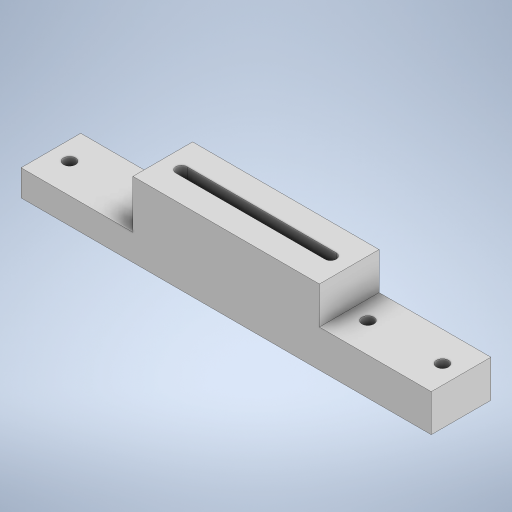
# Autodesk Inventor part: middle_hole
Saved by Autodesk Inventor 2023.1 (Build 271208000, 208)
## iProperties
Created: 2023-11-20
Part Number: middle_hole
Material: Všeobecné
Document SubType Name: Modeling
Designer: zavrel
Density: 1 g/cm^3
Appearance: Výchozí
Author: zavrel
Autodesk Inventor part; units mm, degrees
ref_plane "YZ Plane" through (0, 0, 0) normal (1, 0, 0) x (0, 1, 0)
ref_plane "XZ Plane" through (0, 0, 0) normal (0, 1, 0) x (-1, 0, 0)
ref_plane "XY Plane" through (0, 0, 0) normal (0, 0, 1) x (1, 0, 0)
sketch "Náčrt1" plane through (0, 0, 0) normal (0, 1, 0) x (-1, 0, 0)
  line L0 (0, 0) -> (110, 0)
  line L1 (110, 0) -> (110, -16)
  line L2 (110, -16) -> (0, -16)
  line L3 (0, -16) -> (0, 0)
  line L4 (55, -16) -> (55, 0) construction
  line L5 (110, -8) -> (0, -8) construction
  circle A0 centre (105, -8) radius 1.6
  circle A1 centre (85, -8) radius 1.6
  line L6 (105, -8) -> (105, -2.8731) construction
  line L7 (85, -8) -> (85, -2.8731) construction
  line L8 (105, -5.7373) -> (103.8686, -6.8686)
  line L9 (105, -5.7373) -> (106.1314, -6.8686)
  line L10 (85, -5.7373) -> (83.8686, -6.8686)
  line L11 (85, -5.7373) -> (86.1314, -6.8686)
  circle A2 centre (5, -8) radius 1.6
  circle A3 centre (25, -8) radius 1.6
  line L12 (5, -8) -> (5, -2.8731) construction
  line L13 (25, -8) -> (25, -2.8731) construction
  line L14 (5, -5.7373) -> (6.1314, -6.8686)
  line L15 (5, -5.7373) -> (3.8686, -6.8686)
  line L16 (25, -5.7373) -> (26.1314, -6.8686)
  line L17 (25, -5.7373) -> (23.8686, -6.8686)
  dimension "d0" = 16
  dimension "d1" = 110
  dimension "d4" = 3.2
  dimension "d6" = 25
  dimension "d7" = 5
  dimension "d49" = 90
  dimension "d54" = 90
  constraints: 36 end point, 10 symmetric about line, 4 centre point, 4 midpoint, 4 point on circle, 4 point on line, 2 parallel, 2 tangent, 2 vertical, 1 equal radius, 1 horizontal, 1 perpendicular, 2 other
  measures "d0" distance between parallel lines of L2 L0
  measures "d1" distance of L1.end L2.end
  measures "d4" diameter of A0
  measures "d6" distance from line of L1 L7.start
  measures "d7" distance from line of L1 L6.start
  measures "d49" angle of L9 L8
  measures "d54" angle of L11 L10
extrude "Vysunutí1" add sketch "Náčrt1" along normal blind 20 contours L0 L1 L2 L3 | A0 L8 L9 | A1 L10 L11 | A2 L15 L14 | A3 L17 L16
sketch "Sketch11" plane through (0, 20, 0) normal (0, 1, 0) x (1, 0, 0)
  line L0 (0, 16) -> (-110, 16) projected
  line L1 (-110, 16) -> (-110, 0) projected
  line L2 (-110, 0) -> (0, 0) projected
  line L3 (0, 0) -> (0, 16) projected
  circle A0 centre (-5, 8) radius 1.6 projected
  circle A1 centre (-25, 8) radius 1.6 projected
  circle A2 centre (-85, 8) radius 1.6 projected
  circle A3 centre (-105, 8) radius 1.6 projected
  line L4 (-30, 16) -> (-30, 0)
  line L5 (-110, 0) -> (0, 0) projected
  dimension "d55" = 30
  constraints: 2 end point, 2 point on line, 1 perpendicular
  measures "d55" distance between parallel lines of L3 L4
extrude "Extrusion9" cut sketch "Sketch11" against normal blind 10 contours L3 L2 L4 L0 | A0 | A1
sketch "Sketch12" plane through (0, 20, 0) normal (0, 1, 0) x (1, 0, 0)
  circle A0 centre (-105, 8) radius 1.6 projected
  circle A1 centre (-85, 8) radius 1.6 projected
  line L0 (-30, 0) -> (-30, 16) projected
  line L1 (-30, 16) -> (-110, 16) projected
  line L2 (-110, 16) -> (-110, 0) projected
  line L3 (-110, 0) -> (-30, 0) projected
  line L4 (0, 16) -> (-110, 16) projected
  line L5 (-80, 16) -> (-80, 0)
  line L6 (-110, 0) -> (0, 0) projected
  dimension "d58" = 30
  constraints: 2 end point, 2 point on line, 1 perpendicular
  measures "d58" distance between parallel lines of L5 L2
extrude "Extrusion10" cut sketch "Sketch12" against normal blind 13 contours A0 | A1 | L3 L2 L1 L5
sketch "Sketch13" plane through (0, 0, 0) normal (0, -1, 0) x (1, 0, 0)
  line L0 (0, -16) -> (-110, -16) projected
  line L1 (0, 0) -> (0, -16) projected
  line L2 (-110, 0) -> (0, 0) projected
  line L3 (-110, -16) -> (-110, 0) projected
  circle A0 centre (-5, -8) radius 1.6 projected
  circle A1 centre (-25, -8) radius 1.6 projected
  circle A2 centre (-85, -8) radius 1.6 projected
  circle A3 centre (-105, -8) radius 1.6 projected
  line L4 (-110, -16) -> (-110, 0) construction
  line L5 (-110, -8) -> (0, -8) construction
  line L6 (-75, -8) -> (-35, -8) construction
  line L7 (-75, -9.5) -> (-35, -9.5)
  line L8 (-35, -6.5) -> (-75, -6.5)
  arc A4 (-75, -6.5) -> (-75, -9.5) centre (-75, -8) ccw
  arc A5 (-35, -9.5) -> (-35, -6.5) centre (-35, -8) ccw
  point P0 (-55, -8)
  dimension "d61" = 3
  dimension "d62" = 40
  constraints: 10 end point, 4 midpoint, 4 point on circle, 4 tangent, 2 centre point, 1 parallel, 1 point on line
  measures "d61" distance between parallel lines of L7 L8
  measures "d62" distance of L6.start L6.end
extrude "Extrusion11" cut sketch "Sketch13" against normal through all contours A4 L8 A5 L7
sketch "Sketch14" plane through (0, 0, 0) normal (0, -1, 0) x (1, 0, 0)
  line L0 (-75, -6.5) -> (-35, -6.5) projected
  arc A0 (-35, -9.5) -> (-35, -6.5) centre (-35, -8) ccw projected
  line L1 (-35, -9.5) -> (-75, -9.5) projected
  arc A1 (-75, -6.5) -> (-75, -9.5) centre (-75, -8) ccw projected
  line L2 (0, -16) -> (-110, -16) projected
  line L3 (0, 0) -> (0, -16) projected
  line L4 (-110, 0) -> (0, 0) projected
  line L5 (-110, -16) -> (-110, 0) projected
  circle A2 centre (-5, -8) radius 1.6 projected
  circle A3 centre (-25, -8) radius 1.6 projected
  circle A4 centre (-85, -8) radius 1.6 projected
  circle A5 centre (-105, -8) radius 1.6 projected
  circle A6 centre (-105, -8) radius 1.6 projected
  line L6 (-101.8246, -8) -> (-103.4123, -10.75)
  line L7 (-103.4123, -10.75) -> (-106.5877, -10.75)
  line L8 (-106.5877, -10.75) -> (-108.1754, -8)
  line L9 (-108.1754, -8) -> (-106.5877, -5.25)
  line L10 (-106.5877, -5.25) -> (-103.4123, -5.25)
  line L11 (-103.4123, -5.25) -> (-101.8246, -8)
  line L12 (-81.8246, -8) -> (-83.4123, -10.75)
  line L13 (-83.4123, -10.75) -> (-86.5877, -10.75)
  line L14 (-86.5877, -10.75) -> (-88.1754, -8)
  line L15 (-88.1754, -8) -> (-86.5877, -5.25)
  line L16 (-86.5877, -5.25) -> (-83.4123, -5.25)
  line L17 (-83.4123, -5.25) -> (-81.8246, -8)
  line L18 (-21.8246, -8) -> (-23.4123, -10.75)
  line L19 (-23.4123, -10.75) -> (-26.5877, -10.75)
  line L20 (-26.5877, -10.75) -> (-28.1754, -8)
  line L21 (-28.1754, -8) -> (-26.5877, -5.25)
  line L22 (-26.5877, -5.25) -> (-23.4123, -5.25)
  line L23 (-23.4123, -5.25) -> (-21.8246, -8)
  line L24 (-1.8246, -8) -> (-3.4123, -10.75)
  line L25 (-3.4123, -10.75) -> (-6.5877, -10.75)
  line L26 (-6.5877, -10.75) -> (-8.1754, -8)
  line L27 (-8.1754, -8) -> (-6.5877, -5.25)
  line L28 (-6.5877, -5.25) -> (-3.4123, -5.25)
  line L29 (-3.4123, -5.25) -> (-1.8246, -8)
  point P0 (-106.1314, -6.8686)
  point P1 (-103.8686, -6.8686)
  dimension "d65" = 5.5
  dimension "d66" = 5.5
  dimension "d67" = 5.5
  dimension "d68" = 5.5
  constraints: 48 end point, 1 coincident, 13 other
  measures "d65" distance between parallel lines of L7 L10
  measures "d66" distance between parallel lines of L13 L16
  measures "d67" distance between parallel lines of L19 L22
  measures "d68" distance between parallel lines of L25 L28
extrude "Extrusion12" cut sketch "Sketch14" against normal blind 2 contours A2 | A3 | A4 | A5 | L6 L7 L8 L9 L10 L11 | L12 L13 L14 L15 L16 L17 | L18 L19 L20 L21 L22 L23 | L24 L25 L26 L27 L28 L29
